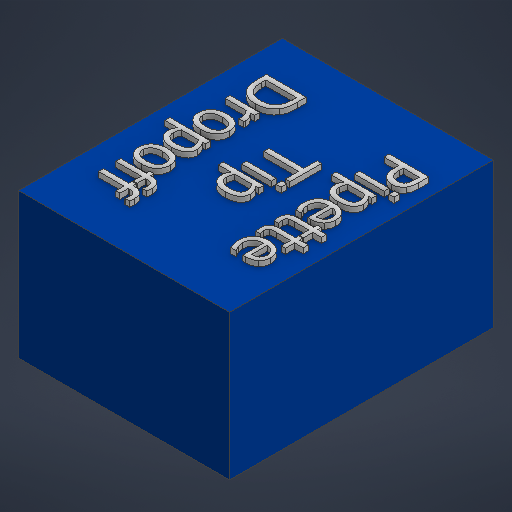
# Autodesk Inventor part: TipDropoff
Saved by Autodesk Inventor 2025.1 (Build 291241000, 241)
## iProperties
Created: 2024-10-04
Part Number: TipDropoff
Material: Generic
Document SubType Name: Modeling
Designer: jerem
Density: 1 g/cm^3
Appearance: Default
Author: jerem
Autodesk Inventor part; units mm, degrees
ref_plane "YZ Plane" through (0, 0, 0) normal (1, 0, 0) x (0, 1, 0)
ref_plane "XZ Plane" through (0, 0, 0) normal (0, 1, 0) x (-1, 0, 0)
ref_plane "XY Plane" through (0, 0, 0) normal (0, 0, 1) x (1, 0, 0)
sketch "Sketch1" plane through (0, 0, 0) normal (0, 1, 0) x (-1, 0, 0)
  line L0 (-40, -50) -> (40, -50)
  line L1 (40, -50) -> (40, 50)
  line L2 (40, 50) -> (-40, 50)
  line L3 (-40, 50) -> (-40, -50)
  line L4 (-40, -50) -> (40, 50) construction
  line L5 (40, -50) -> (-40, 50) construction
  point P0 (0, 0)
  dimension "d0" = 80
  dimension "d1" = 100
  constraints: 12 end point, 2 midpoint, 2 parallel, 1 horizontal, 1 perpendicular
  measures "d0" distance of L2.end L1.end
  measures "d1" distance of L1.end L0.end
extrude "Extrusion1" add sketch "Sketch1" along normal blind 55
sketch "Sketch2" plane through (0, 55, 0) normal (0, 1, 0) x (1, 0, 0)
  line L0 (10.9996, 31.8778) -> (10.9996, -31.3722) construction
  line L1 (10.9996, -31.3722) -> (-8.9113, -31.3722) construction
  line L2 (-8.9113, -31.3722) -> (-8.9113, 31.8778) construction
  line L3 (-8.9113, 31.8778) -> (10.9996, 31.8778) construction
  spline S0 degree 2 poles (30.7433, 20.7593) (29.7709, 20.7593) (28.0205, 21.4522) (27.4127, 22.0721) knots 0 0 0 1 2 2 2
  spline S1 degree 2 poles (27.4127, 22.0721) (26.6469, 22.8501) (25.8568, 24.953) (25.8568, 26.5575) knots 0 0 0 1 2 2 2
  line L4 (25.8568, 26.5575) -> (25.8568, 28.2472)
  line L5 (25.8568, 28.2472) -> (20.2652, 28.2472)
  line L6 (20.2652, 28.2472) -> (20.2652, 30.2407)
  line L7 (20.2652, 30.2407) -> (35.2652, 30.2407)
  line L8 (35.2652, 30.2407) -> (35.2652, 26.4724)
  spline S2 degree 2 poles (35.2652, 26.4724) (35.2652, 25.1353) (34.8276, 23.2634) (34.3292, 22.5462) knots 0 0 0 1 2 2 2
  spline S3 degree 2 poles (34.3292, 22.5462) (33.7579, 21.7075) (31.9953, 20.7593) (30.7433, 20.7593) knots 0 0 0 1 2 2 2
  spline S4 degree 2 poles (30.6825, 22.8379) (31.4605, 22.8379) (32.6031, 23.3728) (32.9678, 23.9198) knots 0 0 0 1 2 2 2
  spline S5 degree 2 poles (32.9678, 23.9198) (33.2838, 24.3938) (33.5391, 25.658) (33.5391, 26.594) knots 0 0 0 1 2 2 2
  line L9 (33.5391, 26.594) -> (33.5391, 28.2472)
  line L10 (33.5391, 28.2472) -> (27.5585, 28.2472)
  line L11 (27.5585, 28.2472) -> (27.5585, 26.8857)
  spline S6 degree 2 poles (27.5585, 26.8857) (27.5585, 25.6702) (27.9475, 24.175) (28.4581, 23.6888) knots 0 0 0 1 2 2 2
  spline S7 degree 2 poles (28.4581, 23.6888) (28.9078, 23.2391) (29.9653, 22.8379) (30.6825, 22.8379) knots 0 0 0 1 2 2 2
  line L12 (20.2652, 17.0762) -> (20.2652, 18.9724)
  line L13 (20.2652, 18.9724) -> (31.5213, 18.9724)
  line L14 (31.5213, 18.9724) -> (31.5213, 17.0762)
  line L15 (31.5213, 17.0762) -> (20.2652, 17.0762)
  line L16 (33.3932, 16.9425) -> (33.3932, 19.094)
  line L17 (33.3932, 19.094) -> (35.3624, 19.094)
  line L18 (35.3624, 19.094) -> (35.3624, 16.9425)
  line L19 (35.3624, 16.9425) -> (33.3932, 16.9425)
  spline S8 degree 2 poles (26.1971, 4.8598) (23.377, 4.8598) (20.0464, 7.5462) (20.0464, 9.6005) knots 0 0 0 1 2 2 2
  spline S9 degree 2 poles (20.0464, 9.6005) (20.0464, 10.4392) (20.4354, 11.7277) (20.8365, 12.3963) knots 0 0 0 1 2 2 2
  line L20 (20.8365, 12.3963) -> (16.1201, 12.3963)
  line L21 (16.1201, 12.3963) -> (16.1201, 14.2925)
  line L22 (16.1201, 14.2925) -> (31.5213, 14.2925)
  line L23 (31.5213, 14.2925) -> (31.5213, 12.3963)
  line L24 (31.5213, 12.3963) -> (30.3422, 12.3963)
  spline S10 degree 2 poles (30.3422, 12.3963) (30.9864, 11.6912) (31.8373, 9.9652) (31.8373, 8.9562) knots 0 0 0 1 2 2 2
  spline S11 degree 2 poles (31.8373, 8.9562) (31.8373, 7.0235) (28.7741, 4.8598) (26.1971, 4.8598) knots 0 0 0 1 2 2 2
  spline S12 degree 2 poles (25.9783, 6.8169) (27.9111, 6.8169) (30.0383, 8.0446) (30.0383, 9.4182) knots 0 0 0 1 2 2 2
  spline S13 degree 2 poles (30.0383, 9.4182) (30.0383, 10.2204) (29.3211, 11.7277) (28.7619, 12.3963) knots 0 0 0 1 2 2 2
  line L25 (28.7619, 12.3963) -> (22.3681, 12.3963)
  spline S14 degree 2 poles (22.3681, 12.3963) (22.0156, 11.6548) (21.7482, 10.5972) (21.7482, 9.9165) knots 0 0 0 1 2 2 2
  spline S15 degree 2 poles (21.7482, 9.9165) (21.7482, 8.4457) (23.9119, 6.8169) (25.9783, 6.8169) knots 0 0 0 1 2 2 2
  spline S16 degree 2 poles (20.0099, -1.9959) (20.0099, 0.7026) (23.0367, 3.6686) (25.8324, 3.6686) knots 0 0 0 1 2 2 2
  spline S17 degree 2 poles (25.8324, 3.6686) (28.5796, 3.6686) (31.8373, 0.7877) (31.8373, -1.534) knots 0 0 0 1 2 2 2
  spline S18 degree 2 poles (31.8373, -1.534) (31.8373, -2.5794) (31.2295, -4.1961) (30.5853, -4.7917) knots 0 0 0 1 2 2 2
  spline S19 degree 2 poles (30.5853, -4.7917) (29.941, -5.3995) (28.0812, -6.0438) (26.732, -6.0438) knots 0 0 0 1 2 2 2
  line L26 (26.732, -6.0438) -> (25.6987, -6.0438)
  line L27 (25.6987, -6.0438) -> (25.6987, 1.748)
  spline S20 degree 2 poles (25.6987, 1.748) (23.7417, 1.748) (21.6631, -0.2212) (21.6631, -1.9716) knots 0 0 0 1 2 2 2
  spline S21 degree 2 poles (21.6631, -1.9716) (21.6631, -2.5916) (21.9427, -3.795) (22.1615, -4.2812) knots 0 0 0 1 2 2 2
  spline S22 degree 2 poles (22.1615, -4.2812) (22.4046, -4.7917) (22.83, -5.4968) (23.0245, -5.7277) knots 0 0 0 1 2 2 2
  line L28 (23.0245, -5.7277) -> (23.0245, -5.8371)
  line L29 (23.0245, -5.8371) -> (20.9581, -5.8371)
  spline S23 degree 2 poles (20.9581, -5.8371) (20.8243, -5.5089) (20.4354, -4.5122) (20.326, -4.1232) knots 0 0 0 1 2 2 2
  spline S24 degree 2 poles (20.326, -4.1232) (20.1679, -3.5762) (20.0099, -2.6767) (20.0099, -1.9959) knots 0 0 0 1 2 2 2
  spline S25 degree 2 poles (27.1453, -4.1961) (27.9111, -4.1718) (29.0294, -3.8558) (29.4062, -3.5519) knots 0 0 0 1 2 2 2
  spline S26 degree 2 poles (29.4062, -3.5519) (29.8316, -3.2237) (30.2814, -2.1904) (30.2814, -1.4246) knots 0 0 0 1 2 2 2
  spline S27 degree 2 poles (30.2814, -1.4246) (30.2814, -0.671) (29.8316, 0.3865) (29.394, 0.8242) knots 0 0 0 1 2 2 2
  spline S28 degree 2 poles (29.394, 0.8242) (28.9443, 1.2496) (27.8624, 1.6872) (27.1453, 1.748) knots 0 0 0 1 2 2 2
  line L30 (27.1453, 1.748) -> (27.1453, -4.1961)
  spline S29 degree 2 poles (20.0464, -11.3679) (20.0464, -9.8241) (21.8089, -8.0859) (23.7174, -8.0859) knots 0 0 0 1 2 2 2
  line L31 (23.7174, -8.0859) -> (29.9532, -8.0859)
  line L32 (29.9532, -8.0859) -> (29.9532, -6.8096)
  line L33 (29.9532, -6.8096) -> (31.5213, -6.8096)
  line L34 (31.5213, -6.8096) -> (31.5213, -8.0859)
  line L35 (31.5213, -8.0859) -> (34.7547, -8.0859)
  line L36 (34.7547, -8.0859) -> (34.7547, -9.9822)
  line L37 (34.7547, -9.9822) -> (31.5213, -9.9822)
  line L38 (31.5213, -9.9822) -> (31.5213, -13.4708)
  line L39 (31.5213, -13.4708) -> (29.9532, -13.4708)
  line L40 (29.9532, -13.4708) -> (29.9532, -9.9822)
  line L41 (29.9532, -9.9822) -> (24.5926, -9.9822)
  spline S30 degree 2 poles (24.5926, -9.9822) (23.7417, -9.9822) (22.8057, -10.0429) (22.4046, -10.2496) knots 0 0 0 1 2 2 2
  spline S31 degree 2 poles (22.4046, -10.2496) (22.0521, -10.4198) (21.6995, -11.1856) (21.6995, -11.842) knots 0 0 0 1 2 2 2
  spline S32 degree 2 poles (21.6995, -11.842) (21.6995, -12.3039) (21.9791, -13.1669) (22.0642, -13.3614) knots 0 0 0 1 2 2 2
  line L42 (22.0642, -13.3614) -> (22.0642, -13.4708)
  line L43 (22.0642, -13.4708) -> (20.3624, -13.4708)
  spline S33 degree 2 poles (20.3624, -13.4708) (20.2166, -12.936) (20.0464, -11.842) (20.0464, -11.3679) knots 0 0 0 1 2 2 2
  spline S34 degree 2 poles (20.0464, -18.2723) (20.0464, -16.7285) (21.8089, -14.9903) (23.7174, -14.9903) knots 0 0 0 1 2 2 2
  line L44 (23.7174, -14.9903) -> (29.9532, -14.9903)
  line L45 (29.9532, -14.9903) -> (29.9532, -13.7139)
  line L46 (29.9532, -13.7139) -> (31.5213, -13.7139)
  line L47 (31.5213, -13.7139) -> (31.5213, -14.9903)
  line L48 (31.5213, -14.9903) -> (34.7547, -14.9903)
  line L49 (34.7547, -14.9903) -> (34.7547, -16.8865)
  line L50 (34.7547, -16.8865) -> (31.5213, -16.8865)
  line L51 (31.5213, -16.8865) -> (31.5213, -20.3752)
  line L52 (31.5213, -20.3752) -> (29.9532, -20.3752)
  line L53 (29.9532, -20.3752) -> (29.9532, -16.8865)
  line L54 (29.9532, -16.8865) -> (24.5926, -16.8865)
  spline S35 degree 2 poles (24.5926, -16.8865) (23.7417, -16.8865) (22.8057, -16.9473) (22.4046, -17.154) knots 0 0 0 1 2 2 2
  spline S36 degree 2 poles (22.4046, -17.154) (22.0521, -17.3241) (21.6995, -18.0899) (21.6995, -18.7464) knots 0 0 0 1 2 2 2
  spline S37 degree 2 poles (21.6995, -18.7464) (21.6995, -19.2083) (21.9791, -20.0713) (22.0642, -20.2658) knots 0 0 0 1 2 2 2
  line L55 (22.0642, -20.2658) -> (22.0642, -20.3752)
  line L56 (22.0642, -20.3752) -> (20.3624, -20.3752)
  spline S38 degree 2 poles (20.3624, -20.3752) (20.2166, -19.8404) (20.0464, -18.7464) (20.0464, -18.2723) knots 0 0 0 1 2 2 2
  spline S39 degree 2 poles (20.0099, -26.6596) (20.0099, -23.9611) (23.0367, -20.9951) (25.8324, -20.9951) knots 0 0 0 1 2 2 2
  spline S40 degree 2 poles (25.8324, -20.9951) (28.5796, -20.9951) (31.8373, -23.876) (31.8373, -26.1977) knots 0 0 0 1 2 2 2
  spline S41 degree 2 poles (31.8373, -26.1977) (31.8373, -27.2431) (31.2295, -28.8598) (30.5853, -29.4554) knots 0 0 0 1 2 2 2
  spline S42 degree 2 poles (30.5853, -29.4554) (29.941, -30.0632) (28.0812, -30.7075) (26.732, -30.7075) knots 0 0 0 1 2 2 2
  line L57 (26.732, -30.7075) -> (25.6987, -30.7075)
  line L58 (25.6987, -30.7075) -> (25.6987, -22.9157)
  spline S43 degree 2 poles (25.6987, -22.9157) (23.7417, -22.9157) (21.6631, -24.8849) (21.6631, -26.6353) knots 0 0 0 1 2 2 2
  spline S44 degree 2 poles (21.6631, -26.6353) (21.6631, -27.2553) (21.9427, -28.4587) (22.1615, -28.9449) knots 0 0 0 1 2 2 2
  spline S45 degree 2 poles (22.1615, -28.9449) (22.4046, -29.4554) (22.83, -30.1605) (23.0245, -30.3914) knots 0 0 0 1 2 2 2
  line L59 (23.0245, -30.3914) -> (23.0245, -30.5008)
  line L60 (23.0245, -30.5008) -> (20.9581, -30.5008)
  spline S46 degree 2 poles (20.9581, -30.5008) (20.8243, -30.1726) (20.4354, -29.1758) (20.326, -28.7869) knots 0 0 0 1 2 2 2
  spline S47 degree 2 poles (20.326, -28.7869) (20.1679, -28.2399) (20.0099, -27.3404) (20.0099, -26.6596) knots 0 0 0 1 2 2 2
  spline S48 degree 2 poles (27.1453, -28.8598) (27.9111, -28.8355) (29.0294, -28.5194) (29.4062, -28.2156) knots 0 0 0 1 2 2 2
  spline S49 degree 2 poles (29.4062, -28.2156) (29.8316, -27.8874) (30.2814, -26.8541) (30.2814, -26.0883) knots 0 0 0 1 2 2 2
  spline S50 degree 2 poles (30.2814, -26.0883) (30.2814, -25.3347) (29.8316, -24.2771) (29.394, -23.8395) knots 0 0 0 1 2 2 2
  spline S51 degree 2 poles (29.394, -23.8395) (28.9443, -23.4141) (27.8624, -22.9765) (27.1453, -22.9157) knots 0 0 0 1 2 2 2
  line L61 (27.1453, -22.9157) -> (27.1453, -28.8598)
  line L62 (-4.4319, 9.3148) -> (8.7934, 9.3148)
  line L63 (8.7934, 9.3148) -> (8.7934, 14.3472)
  line L64 (8.7934, 14.3472) -> (10.5681, 14.3472)
  line L65 (10.5681, 14.3472) -> (10.5681, 2.2889)
  line L66 (10.5681, 2.2889) -> (8.7934, 2.2889)
  line L67 (8.7934, 2.2889) -> (8.7934, 7.3213)
  line L68 (8.7934, 7.3213) -> (-4.4319, 7.3213)
  line L69 (-4.4319, 7.3213) -> (-4.4319, 9.3148)
  line L70 (-4.4319, -1.0174) -> (-4.4319, 0.8789)
  line L71 (-4.4319, 0.8789) -> (6.8242, 0.8789)
  line L72 (6.8242, 0.8789) -> (6.8242, -1.0174)
  line L73 (6.8242, -1.0174) -> (-4.4319, -1.0174)
  line L74 (8.6961, -1.1511) -> (8.6961, 1.0004)
  line L75 (8.6961, 1.0004) -> (10.6653, 1.0004)
  line L76 (10.6653, 1.0004) -> (10.6653, -1.1511)
  line L77 (10.6653, -1.1511) -> (8.6961, -1.1511)
  spline S52 degree 2 poles (1.5, -13.2338) (-1.3201, -13.2338) (-4.6507, -10.5474) (-4.6507, -8.4931) knots 0 0 0 1 2 2 2
  spline S53 degree 2 poles (-4.6507, -8.4931) (-4.6507, -7.6544) (-4.2617, -6.3659) (-3.8606, -5.6973) knots 0 0 0 1 2 2 2
  line L78 (-3.8606, -5.6973) -> (-8.577, -5.6973)
  line L79 (-8.577, -5.6973) -> (-8.577, -3.8011)
  line L80 (-8.577, -3.8011) -> (6.8242, -3.8011)
  line L81 (6.8242, -3.8011) -> (6.8242, -5.6973)
  line L82 (6.8242, -5.6973) -> (5.6451, -5.6973)
  spline S54 degree 2 poles (5.6451, -5.6973) (6.2893, -6.4023) (7.1402, -8.1284) (7.1402, -9.1374) knots 0 0 0 1 2 2 2
  spline S55 degree 2 poles (7.1402, -9.1374) (7.1402, -11.0701) (4.077, -13.2338) (1.5, -13.2338) knots 0 0 0 1 2 2 2
  spline S56 degree 2 poles (1.2812, -11.2767) (3.2139, -11.2767) (5.3412, -10.049) (5.3412, -8.6754) knots 0 0 0 1 2 2 2
  spline S57 degree 2 poles (5.3412, -8.6754) (5.3412, -7.8732) (4.624, -6.3659) (4.0648, -5.6973) knots 0 0 0 1 2 2 2
  line L83 (4.0648, -5.6973) -> (-2.329, -5.6973)
  spline S58 degree 2 poles (-2.329, -5.6973) (-2.6815, -6.4388) (-2.9489, -7.4964) (-2.9489, -8.1771) knots 0 0 0 1 2 2 2
  spline S59 degree 2 poles (-2.9489, -8.1771) (-2.9489, -9.6479) (-0.7852, -11.2767) (1.2812, -11.2767) knots 0 0 0 1 2 2 2
  spline S60 degree 2 poles (-21.6412, 21.3002) (-23.6955, 21.3002) (-27.0018, 22.9656) (-27.9256, 24.3635) knots 0 0 0 1 2 2 2
  spline S61 degree 2 poles (-27.9256, 24.3635) (-28.6428, 25.5061) (-29.129, 27.8521) (-29.129, 29.6754) knots 0 0 0 1 2 2 2
  line L84 (-29.129, 29.6754) -> (-29.129, 33.1276)
  line L85 (-29.129, 33.1276) -> (-14.129, 33.1276)
  line L86 (-14.129, 33.1276) -> (-14.129, 29.7119)
  spline S62 degree 2 poles (-14.129, 29.7119) (-14.129, 27.5968) (-14.7611, 25.19) (-15.3203, 24.3391) knots 0 0 0 1 2 2 2
  spline S63 degree 2 poles (-15.3203, 24.3391) (-16.2806, 22.8926) (-19.4532, 21.3002) (-21.6412, 21.3002) knots 0 0 0 1 2 2 2
  spline S64 degree 2 poles (-21.6169, 23.3789) (-19.8908, 23.3789) (-17.4475, 24.5215) (-16.7546, 25.6519) knots 0 0 0 1 2 2 2
  spline S65 degree 2 poles (-16.7546, 25.6519) (-16.2806, 26.4542) (-15.8551, 28.2654) (-15.8551, 29.6147) knots 0 0 0 1 2 2 2
  line L87 (-15.8551, 29.6147) -> (-15.8551, 31.1341)
  line L88 (-15.8551, 31.1341) -> (-27.4029, 31.1341)
  line L89 (-27.4029, 31.1341) -> (-27.4029, 29.6147)
  spline S66 degree 2 poles (-27.4029, 29.6147) (-27.4029, 28.2897) (-26.9775, 26.284) (-26.4062, 25.4696) knots 0 0 0 1 2 2 2
  spline S67 degree 2 poles (-26.4062, 25.4696) (-25.7011, 24.4242) (-23.3673, 23.3789) (-21.6169, 23.3789) knots 0 0 0 1 2 2 2
  line L90 (-19.9029, 13.314) -> (-19.9029, 13.4113)
  spline S68 degree 2 poles (-19.9029, 13.4113) (-19.8422, 13.6301) (-19.8178, 14.1041) (-19.8178, 14.4323) knots 0 0 0 1 2 2 2
  spline S69 degree 2 poles (-19.8178, 14.4323) (-19.8178, 15.1981) (-20.4864, 16.7054) (-21.1428, 17.3861) knots 0 0 0 1 2 2 2
  line L91 (-21.1428, 17.3861) -> (-29.129, 17.3861)
  line L92 (-29.129, 17.3861) -> (-29.129, 19.2824)
  line L93 (-29.129, 19.2824) -> (-17.8729, 19.2824)
  line L94 (-17.8729, 19.2824) -> (-17.8729, 17.3861)
  line L95 (-17.8729, 17.3861) -> (-19.5504, 17.3861)
  spline S70 degree 2 poles (-19.5504, 17.3861) (-18.6266, 16.3529) (-17.8729, 14.8092) (-17.8729, 14.0798) knots 0 0 0 1 2 2 2
  spline S71 degree 2 poles (-17.8729, 14.0798) (-17.8729, 13.7881) (-17.8973, 13.4964) (-17.9337, 13.314) knots 0 0 0 1 2 2 2
  line L96 (-17.9337, 13.314) -> (-19.9029, 13.314)
  spline S72 degree 2 poles (-23.501, 2.5928) (-26.3454, 2.5928) (-29.4451, 5.3278) (-29.4451, 7.613) knots 0 0 0 1 2 2 2
  spline S73 degree 2 poles (-29.4451, 7.613) (-29.4451, 9.9591) (-26.2482, 12.6455) (-23.501, 12.6455) knots 0 0 0 1 2 2 2
  spline S74 degree 2 poles (-23.501, 12.6455) (-20.6809, 12.6455) (-17.5569, 9.874) (-17.5569, 7.613) knots 0 0 0 1 2 2 2
  spline S75 degree 2 poles (-17.5569, 7.613) (-17.5569, 5.3278) (-20.6687, 2.5928) (-23.501, 2.5928) knots 0 0 0 1 2 2 2
  spline S76 degree 2 poles (-23.501, 4.5498) (-21.313, 4.5498) (-19.1858, 6.1422) (-19.1858, 7.613) knots 0 0 0 1 2 2 2
  spline S77 degree 2 poles (-19.1858, 7.613) (-19.1858, 9.0839) (-21.313, 10.6884) (-23.501, 10.6884) knots 0 0 0 1 2 2 2
  spline S78 degree 2 poles (-23.501, 10.6884) (-25.6282, 10.6884) (-27.8162, 9.0839) (-27.8162, 7.613) knots 0 0 0 1 2 2 2
  spline S79 degree 2 poles (-27.8162, 7.613) (-27.8162, 6.1544) (-25.6647, 4.5498) (-23.501, 4.5498) knots 0 0 0 1 2 2 2
  spline S80 degree 2 poles (-23.1971, -8.7848) (-26.0172, -8.7848) (-29.3478, -6.0985) (-29.3478, -4.0442) knots 0 0 0 1 2 2 2
  spline S81 degree 2 poles (-29.3478, -4.0442) (-29.3478, -3.2054) (-28.9588, -1.9169) (-28.5577, -1.2484) knots 0 0 0 1 2 2 2
  line L97 (-28.5577, -1.2484) -> (-33.2741, -1.2484)
  line L98 (-33.2741, -1.2484) -> (-33.2741, 0.6479)
  line L99 (-33.2741, 0.6479) -> (-17.8729, 0.6479)
  line L100 (-17.8729, 0.6479) -> (-17.8729, -1.2484)
  line L101 (-17.8729, -1.2484) -> (-19.052, -1.2484)
  spline S82 degree 2 poles (-19.052, -1.2484) (-18.4078, -1.9534) (-17.5569, -3.6795) (-17.5569, -4.6884) knots 0 0 0 1 2 2 2
  spline S83 degree 2 poles (-17.5569, -4.6884) (-17.5569, -6.6211) (-20.6201, -8.7848) (-23.1971, -8.7848) knots 0 0 0 1 2 2 2
  spline S84 degree 2 poles (-23.4159, -6.8278) (-21.4832, -6.8278) (-19.3559, -5.6001) (-19.3559, -4.2265) knots 0 0 0 1 2 2 2
  spline S85 degree 2 poles (-19.3559, -4.2265) (-19.3559, -3.4242) (-20.0731, -1.9169) (-20.6323, -1.2484) knots 0 0 0 1 2 2 2
  line L102 (-20.6323, -1.2484) -> (-27.0261, -1.2484)
  spline S86 degree 2 poles (-27.0261, -1.2484) (-27.3786, -1.9899) (-27.646, -3.0474) (-27.646, -3.7281) knots 0 0 0 1 2 2 2
  spline S87 degree 2 poles (-27.646, -3.7281) (-27.646, -5.1989) (-25.4823, -6.8278) (-23.4159, -6.8278) knots 0 0 0 1 2 2 2
  spline S88 degree 2 poles (-23.501, -20.0045) (-26.3454, -20.0045) (-29.4451, -17.2694) (-29.4451, -14.9842) knots 0 0 0 1 2 2 2
  spline S89 degree 2 poles (-29.4451, -14.9842) (-29.4451, -12.6382) (-26.2482, -9.9518) (-23.501, -9.9518) knots 0 0 0 1 2 2 2
  spline S90 degree 2 poles (-23.501, -9.9518) (-20.6809, -9.9518) (-17.5569, -12.7233) (-17.5569, -14.9842) knots 0 0 0 1 2 2 2
  spline S91 degree 2 poles (-17.5569, -14.9842) (-17.5569, -17.2694) (-20.6687, -20.0045) (-23.501, -20.0045) knots 0 0 0 1 2 2 2
  spline S92 degree 2 poles (-23.501, -18.0474) (-21.313, -18.0474) (-19.1858, -16.455) (-19.1858, -14.9842) knots 0 0 0 1 2 2 2
  spline S93 degree 2 poles (-19.1858, -14.9842) (-19.1858, -13.5134) (-21.313, -11.9088) (-23.501, -11.9088) knots 0 0 0 1 2 2 2
  spline S94 degree 2 poles (-23.501, -11.9088) (-25.6282, -11.9088) (-27.8162, -13.5134) (-27.8162, -14.9842) knots 0 0 0 1 2 2 2
  spline S95 degree 2 poles (-27.8162, -14.9842) (-27.8162, -16.4429) (-25.6647, -18.0474) (-23.501, -18.0474) knots 0 0 0 1 2 2 2
  line L103 (-15.2838, -27.8691) -> (-15.2838, -27.7719)
  spline S96 degree 2 poles (-15.2838, -27.7719) (-15.1866, -27.5166) (-15.0164, -26.5685) (-15.0164, -26.1917) knots 0 0 0 1 2 2 2
  spline S97 degree 2 poles (-15.0164, -26.1917) (-15.0164, -25.0004) (-16.0861, -23.9793) (-17.4961, -23.9793) knots 0 0 0 1 2 2 2
  line L104 (-17.4961, -23.9793) -> (-17.8729, -23.9793)
  line L105 (-17.8729, -23.9793) -> (-17.8729, -27.1155)
  line L106 (-17.8729, -27.1155) -> (-19.441, -27.1155)
  line L107 (-19.441, -27.1155) -> (-19.441, -24.0401)
  line L108 (-19.441, -24.0401) -> (-29.129, -24.0401)
  line L109 (-29.129, -24.0401) -> (-29.129, -22.1438)
  line L110 (-29.129, -22.1438) -> (-19.441, -22.1438)
  line L111 (-19.441, -22.1438) -> (-19.441, -20.8675)
  line L112 (-19.441, -20.8675) -> (-17.8729, -20.8675)
  line L113 (-17.8729, -20.8675) -> (-17.8729, -22.1438)
  line L114 (-17.8729, -22.1438) -> (-17.4961, -22.1438)
  spline S98 degree 2 poles (-17.4961, -22.1438) (-15.4783, -22.1438) (-13.3632, -24.1009) (-13.3632, -25.9242) knots 0 0 0 1 2 2 2
  spline S99 degree 2 poles (-13.3632, -25.9242) (-13.3632, -26.4469) (-13.4726, -27.4558) (-13.5456, -27.8691) knots 0 0 0 1 2 2 2
  line L115 (-13.5456, -27.8691) -> (-15.2838, -27.8691)
  line L116 (-15.2838, -34.4331) -> (-15.2838, -34.3359)
  spline S100 degree 2 poles (-15.2838, -34.3359) (-15.1866, -34.0806) (-15.0164, -33.1325) (-15.0164, -32.7557) knots 0 0 0 1 2 2 2
  spline S101 degree 2 poles (-15.0164, -32.7557) (-15.0164, -31.5644) (-16.0861, -30.5434) (-17.4961, -30.5434) knots 0 0 0 1 2 2 2
  line L117 (-17.4961, -30.5434) -> (-17.8729, -30.5434)
  line L118 (-17.8729, -30.5434) -> (-17.8729, -33.6795)
  line L119 (-17.8729, -33.6795) -> (-19.441, -33.6795)
  line L120 (-19.441, -33.6795) -> (-19.441, -30.6041)
  line L121 (-19.441, -30.6041) -> (-29.129, -30.6041)
  line L122 (-29.129, -30.6041) -> (-29.129, -28.7079)
  line L123 (-29.129, -28.7079) -> (-19.441, -28.7079)
  line L124 (-19.441, -28.7079) -> (-19.441, -27.4315)
  line L125 (-19.441, -27.4315) -> (-17.8729, -27.4315)
  line L126 (-17.8729, -27.4315) -> (-17.8729, -28.7079)
  line L127 (-17.8729, -28.7079) -> (-17.4961, -28.7079)
  spline S102 degree 2 poles (-17.4961, -28.7079) (-15.4783, -28.7079) (-13.3632, -30.6649) (-13.3632, -32.4882) knots 0 0 0 1 2 2 2
  spline S103 degree 2 poles (-13.3632, -32.4882) (-13.3632, -33.0109) (-13.4726, -34.0199) (-13.5456, -34.4331) knots 0 0 0 1 2 2 2
  line L128 (-13.5456, -34.4331) -> (-15.2838, -34.4331)
  point P0 (0, 0)
  constraints: 2 other
extrude "Extrusion2" add sketch "Sketch2" along normal blind 2
body "Solid1"
